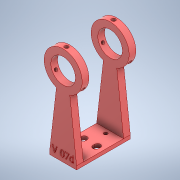
# Autodesk Inventor part: finderMainPartV07
Saved by Autodesk Inventor 2021.1 (Build 251245000, 245)
## iProperties
Created: 2020-06-05
Part Number: finderMainPartV07
Material: PC/ABS Plastic
Document SubType Name: Modeling
Designer: robst
Density: 0.357273 g/cm^3
Appearance: Smooth - Red
Author: robst
Autodesk Inventor part; units mm, degrees
ref_plane "YZ Plane" through (0, 0, 0) normal (1, 0, 0) x (0, 1, 0)
ref_plane "XY Plane" through (0, 0, 0) normal (0, 0, 1) x (1, 0, 0)
sketch "Sketch1" plane through (0, 0, 0) normal (0, 0, 1) x (1, 0, 0)
  arc A0 (19.05, 73.7803) -> (-19.05, 73.7803) centre (0, 0) ccw
  line L0 (0, 86.4803) -> (19.05, 86.4803)
  line L1 (19.05, 86.4803) -> (19.05, 73.7803)
  line L2 (0, 76.2) -> (0, 86.4803) construction
  line L3 (0, 86.4803) -> (-19.05, 86.4803)
  line L4 (-19.05, 86.4803) -> (-19.05, 73.7803)
  dimension "d0" = 152.4
  dimension "d1" = 19.05
  dimension "d2" = 12.7
  constraints: 10 end point, 3 point on circle, 2 symmetric about line, 1 centre point, 1 coincident, 1 horizontal, 1 perpendicular, 1 vertical
  measures "d0" diameter of A0
  measures "d1" distance of L0.start L0.end
  measures "d2" distance of L0.end L1.end
extrude "Extrusion1" add sketch "Sketch1" along normal mid plane 76.2
sketch "Sketch2" plane through (-19.05, 86.4803, 38.1) normal (0, 1, 0) x (1, 0, 0)
  line L0 (0, 76.2) -> (0, 0) construction
  line L1 (0, 38.1) -> (38.1, 38.1) construction
  line L2 (38.1, 76.2) -> (38.1, 0) construction
  line L3 (0, 76.2) -> (38.1, 76.2) construction
  line L4 (19.05, 76.2) -> (19.05, 0) construction
  line L5 (38.1, 0) -> (0, 0) construction
  line L6 (28.575, 36.1585) -> (28.575, 40.0415) construction
  line L7 (23.495, 38.1) -> (23.495, 38.1)
  line L8 (33.655, 38.1) -> (33.655, 38.1)
  line L9 (14.605, 38.1) -> (14.605, 38.1)
  line L10 (4.445, 38.1) -> (4.445, 38.1)
  line L11 (28.575, 39.37) -> (28.575, 36.83) construction
  line L12 (24.4475, 39.37) -> (24.4475, 36.83)
  line L13 (32.7025, 36.83) -> (32.7025, 39.37)
  arc A0 (32.7025, 39.37) -> (24.4475, 39.37) centre (28.575, 39.37) ccw
  arc A1 (24.4475, 36.83) -> (32.7025, 36.83) centre (28.575, 36.83) ccw
  line L14 (13.6525, 39.37) -> (13.6525, 36.83)
  line L15 (5.3975, 36.83) -> (5.3975, 39.37)
  arc A2 (13.6525, 39.37) -> (5.3975, 39.37) centre (9.525, 39.37) ccw
  arc A3 (5.3975, 36.83) -> (13.6525, 36.83) centre (9.525, 36.83) ccw
  point P0 (19.05, 38.1)
  point P1 (28.575, 38.1)
  dimension "d202" = 8.255
  dimension "d204" = 2.54
  constraints: 28 end point, 10 symmetric about line, 8 point on circle, 6 midpoint, 4 centre point, 4 tangent, 2 parallel, 2 perpendicular, 1 point on line, 2 other
  measures "d202" distance between parallel lines of L13 L12
  measures "d204" distance of L11.end L11.start
extrude "Extrusion2" cut sketch "Sketch2" against normal through all
ref_plane "Work Plane1" through (19.05, 73.7803, 38.1) normal (0, 1, 0) x (-1, 0, 0)
sketch "Sketch5" plane through (0, 0, 38.1) normal (0, 0, 1) x (1, 0, 0)
  circle A0 centre (0, 193.7953) radius 17.4625
  arc A1 (9.525, 168.5446) -> (-9.525, 168.5446) centre (0, 193.7953) ccw
  arc A2 (19.05, 73.7803) -> (-19.05, 73.7803) centre (0, 0) ccw construction
  line L0 (-19.05, 73.7803) -> (19.05, 73.7803) construction
  line L1 (19.05, 86.4803) -> (9.525, 168.5446)
  line L2 (19.05, 86.4803) -> (-19.05, 86.4803) construction
  line L3 (0, 86.4803) -> (0, 193.7953) construction
  line L4 (-19.05, 86.4803) -> (-9.525, 168.5446)
  line L5 (-19.05, 86.4803) -> (19.05, 86.4803)
  dimension "d15" = 34.925
  dimension "d16" = 9.525
  dimension "d17" = 120.015
  dimension "d18" = 9.525
  constraints: 10 end point, 2 centre point, 2 horizontal, 2 point on circle, 1 coincident, 1 midpoint, 1 perpendicular, 1 symmetric about line
  measures "d15" diameter of A0
  measures "d16" radial gap between concentric circles of A1 A0
  measures "d17" distance from line of A0.centre L0
  measures "d18" distance from line of L1.end L3
extrude "Extrusion4" add sketch "Sketch5" against normal blind 9.525
ref_plane "Work Plane2" through (0, 220.7828, 38.1) normal (0, 1, 0) x (-1, 0, 0)
sketch "Sketch6" plane through (0, 220.7828, 38.1) normal (0, 1, 0) x (-1, 0, 0)
  line L0 (-26.9875, -9.525) -> (26.9875, -9.525) projected
  line L1 (26.9875, 0) -> (26.9875, -9.525) projected
  line L2 (26.9875, 0) -> (26.9875, -9.525) construction
  line L3 (26.9875, -4.7625) -> (-26.9875, -4.7625) construction
  line L4 (-26.9875, 0) -> (-26.9875, -9.525) construction
  point P0 (0, -38.1)
  point P1 (9.525, -9.525)
  point P2 (-9.525, -9.525)
  point P3 (0, -4.7625)
  constraints: 3 midpoint, 2 end point
hole "Hole2" at (0, 220.7828, 33.3375) direction (0, -1, 0) diameter 4.4958 depth 10.16 tip angle 118 counterbore diameter 5.6134 counterbore depth 6.35 clearance for "Hex Machine Screw" size "#8" standard "Ansi Unified Screw Threads"
sketch "Sketch20" plane through (19.05, 73.7803, 38.1) normal (1, 0, 0) x (0, 0, -1)
  line L0 (0, 12.7) -> (0, 0) projected
  line L1 (76.2, 12.7) -> (76.2, 0) projected
  line L2 (0, 0) -> (76.2, 0)
  line L3 (76.2, 0) -> (76.2, 6.35)
  line L4 (76.2, 6.35) -> (0, 6.35)
  line L5 (0, 6.35) -> (0, 0)
  point P0 (38.1, -73.7803)
  point P1 (0, 6.35)
  constraints: 8 end point, 2 parallel, 1 horizontal, 1 midpoint, 1 perpendicular
extrude "Extrusion7" cut sketch "Sketch20" against normal through all
sketch "Sketch22" plane through (-19.05, 86.4803, 28.575) normal (0, 1, 0) x (1, 0, 0)
  line L0 (46.0375, 0) -> (-7.9375, 0) projected
  line L1 (44.45, 57.15) -> (-6.35, 57.15) projected
  line L2 (-6.35, 66.675) -> (44.45, 66.675) projected
  point P0 (19.05, 28.575)
  point P1 (19.05, 6.35)
  point P2 (19.05, 50.8)
  point P3 (9.525, 0)
  point P4 (28.575, 0)
  point P5 (9.525, 57.15)
  point P6 (28.575, 57.15)
  point P7 (28.575, 66.675)
  point P8 (9.525, 66.675)
  dimension "d173" = 6.35
  dimension "d174" = 6.35
  dimension "d183" = 15.875
  measures "d173" distance from line of point (19.05, 6.35) L0
  measures "d174" distance from line of point (19.05, 50.8) L1
  measures "d183" distance from line of point (19.05, 50.8) L2
hole "Hole1" at (0, 86.4803, 22.225) at (0, 86.4803, -22.225) direction (0, -1, 0) diameter 5.1054 end through all clearance for "Socket Head Cap Screw" size "#10" standard "Ansi Unified Screw Threads"
sketch "Sketch23" plane through (19.05, 86.4803, 38.1) normal (1, 0, 0) x (0, 0, -1)
  line L0 (76.2, -6.35) -> (76.2, 0) projected
  line L1 (0, -6.35) -> (76.2, -6.35)
  line L2 (76.2, -6.35) -> (76.2, -5.08)
  line L3 (76.2, -5.08) -> (0, -5.08)
  line L4 (0, -5.08) -> (0, -6.35)
  point P0 (38.1, -86.4803)
  dimension "d185" = 1.27
  constraints: 8 end point, 2 parallel, 1 horizontal, 1 perpendicular, 1 point on line
  measures "d185" distance of L2.end L1.end
extrude "Extrusion8" cut sketch "Sketch23" against normal through all
pattern_circular "Circular Pattern2" count 3 over 360 about axis through (0, 193.7953, 38.1) along (0, 0, -1) of "Hole2"
mirror "Mirror2" about plane through (0, 0, 0) normal (0, 0, 1) of "Extrusion4", "Hole2", "Circular Pattern2"
sketch "Sketch24" plane through (0, 0, 38.1) normal (0, 0, 1) x (1, 0, 0)
  line L0 (-19.05, 86.4803) -> (-9.525, 168.5446) construction
  line L1 (-18.4604, 91.5603) -> (18.4604, 91.5603) construction
  line L2 (9.525, 168.5446) -> (19.05, 86.4803) construction
  line L3 (-19.05, 81.4003) -> (19.05, 81.4003) construction
  line L4 (-8.2596, 96.0053) -> (-11.3214, 87.1153)
  line L5 (-11.3214, 87.1153) -> (-12.5966, 87.1153)
  line L6 (-12.5966, 87.1153) -> (-15.6584, 96.0053)
  line L7 (-15.6584, 96.0053) -> (-14.3904, 96.0053)
  line L8 (-14.3904, 96.0053) -> (-11.9266, 88.621)
  line L9 (-11.9266, 88.621) -> (-9.4627, 96.0053)
  line L10 (-9.4627, 96.0053) -> (-8.2596, 96.0053)
  spline S0 degree 2 poles (1.7902, 91.5603) (1.7902, 89.1685) (0.3998, 86.928) (-1.0482, 86.928) knots 0 0 0 1 2 2 2
  spline S1 degree 2 poles (-1.0482, 86.928) (-2.5179, 86.928) (-3.8939, 89.2118) (-3.8939, 91.5531) knots 0 0 0 1 2 2 2
  spline S2 degree 2 poles (-3.8939, 91.5531) (-3.8939, 93.9593) (-2.5035, 96.1854) (-1.0482, 96.1854) knots 0 0 0 1 2 2 2
  spline S3 degree 2 poles (-1.0482, 96.1854) (0.4142, 96.1854) (1.7902, 93.8801) (1.7902, 91.5603) knots 0 0 0 1 2 2 2
  spline S4 degree 2 poles (0.263, 88.8515) (0.4359, 89.291) (0.5799, 90.6454) (0.5799, 91.5603) knots 0 0 0 1 2 2 2
  spline S5 degree 2 poles (0.5799, 91.5603) (0.5799, 92.4753) (0.4359, 93.8225) (0.2557, 94.2763) knots 0 0 0 1 2 2 2
  spline S6 degree 2 poles (0.2557, 94.2763) (0.0756, 94.7302) (-0.5511, 95.1985) (-1.0482, 95.1985) knots 0 0 0 1 2 2 2
  spline S7 degree 2 poles (-1.0482, 95.1985) (-1.5453, 95.1985) (-2.1865, 94.7302) (-2.3738, 94.2619) knots 0 0 0 1 2 2 2
  spline S8 degree 2 poles (-2.3738, 94.2619) (-2.5539, 93.808) (-2.6836, 92.4248) (-2.6836, 91.5531) knots 0 0 0 1 2 2 2
  spline S9 degree 2 poles (-2.6836, 91.5531) (-2.6836, 90.6166) (-2.5683, 89.363) (-2.381, 88.8732) knots 0 0 0 1 2 2 2
  spline S10 degree 2 poles (-2.381, 88.8732) (-2.2081, 88.4121) (-1.5669, 87.915) (-1.0482, 87.915) knots 0 0 0 1 2 2 2
  spline S11 degree 2 poles (-1.0482, 87.915) (-0.5583, 87.915) (0.0828, 88.3833) (0.263, 88.8515) knots 0 0 0 1 2 2 2
  line L11 (8.5118, 94.6726) -> (4.6647, 87.1153)
  line L12 (4.6647, 87.1153) -> (3.3968, 87.1153)
  line L13 (3.3968, 87.1153) -> (7.46, 94.9607)
  line L14 (7.46, 94.9607) -> (2.8709, 94.9607)
  line L15 (2.8709, 94.9607) -> (2.8709, 96.0053)
  line L16 (2.8709, 96.0053) -> (8.5118, 96.0053)
  line L17 (8.5118, 96.0053) -> (8.5118, 94.6726)
  line L18 (14.8947, 87.1153) -> (13.7709, 87.1153)
  line L19 (13.7709, 87.1153) -> (13.7709, 87.7925)
  spline S12 degree 2 poles (13.7709, 87.7925) (13.5115, 87.5764) (13.1297, 87.2882) (12.8703, 87.1658) knots 0 0 0 1 2 2 2
  spline S13 degree 2 poles (12.8703, 87.1658) (12.6326, 87.0505) (12.1211, 86.928) (11.7825, 86.928) knots 0 0 0 1 2 2 2
  spline S14 degree 2 poles (11.7825, 86.928) (11.235, 86.928) (10.3128, 87.3819) (9.9886, 87.8213) knots 0 0 0 1 2 2 2
  spline S15 degree 2 poles (9.9886, 87.8213) (9.6645, 88.2608) (9.3042, 89.5576) (9.3042, 90.4005) knots 0 0 0 1 2 2 2
  spline S16 degree 2 poles (9.3042, 90.4005) (9.3042, 91.2794) (9.7581, 92.5617) (10.1543, 93.0444) knots 0 0 0 1 2 2 2
  spline S17 degree 2 poles (10.1543, 93.0444) (10.5218, 93.4767) (11.552, 93.9737) (12.1211, 93.9737) knots 0 0 0 1 2 2 2
  spline S18 degree 2 poles (12.1211, 93.9737) (12.6182, 93.9737) (13.3602, 93.7504) (13.7709, 93.5199) knots 0 0 0 1 2 2 2
  line L20 (13.7709, 93.5199) -> (13.7709, 96.4016)
  line L21 (13.7709, 96.4016) -> (14.8947, 96.4016)
  line L22 (14.8947, 96.4016) -> (14.8947, 87.1153)
  line L23 (13.7709, 88.7363) -> (13.7709, 92.5905)
  spline S19 degree 2 poles (13.7709, 92.5905) (13.353, 92.7923) (12.6902, 92.9435) (12.3084, 92.9435) knots 0 0 0 1 2 2 2
  spline S20 degree 2 poles (12.3084, 92.9435) (11.4439, 92.9435) (10.4641, 91.6468) (10.4641, 90.4221) knots 0 0 0 1 2 2 2
  spline S21 degree 2 poles (10.4641, 90.4221) (10.4641, 89.2406) (11.2134, 87.9942) (12.0418, 87.9942) knots 0 0 0 1 2 2 2
  spline S22 degree 2 poles (12.0418, 87.9942) (12.4813, 87.9942) (13.3746, 88.3977) (13.7709, 88.7363) knots 0 0 0 1 2 2 2
  point P0 (0, 0)
  dimension "d198" = 10.16
  constraints: 2 end point, 2 horizontal, 2 point on line
  measures "d198" distance between parallel lines of L1 L3
extrude "Extrusion9" cut sketch "Sketch24" against normal blind 1.27
equation "\"d51\" = 0.125 * Sketch8_Pitch"
equation "\"Sketch8_Pitch\" = 0.79375"
equation "\"d53\" = 60deg"
equation "\"d72\" = 0.125 * Sketch10_Pitch"
equation "\"Sketch10_Pitch\" = 0.79375"
equation "\"d74\" = 60deg"
equation "\"d93\" = 0.125 * Sketch12_Pitch"
equation "\"Sketch12_Pitch\" = 0.79375"
equation "\"d95\" = 60deg"
equation "\"d114\" = 0.125 * Sketch14_Pitch"
equation "\"Sketch14_Pitch\" = 0.79375"
equation "\"d116\" = 60deg"
equation "\"d135\" = 0.125 * Sketch16_Pitch"
equation "\"Sketch16_Pitch\" = 0.79375"
equation "\"d137\" = 60deg"
equation "\"d156\" = 0.125 * Sketch18_Pitch"
equation "\"Sketch18_Pitch\" = 0.79375"
equation "\"d158\" = 60deg"
body "Solid1"
